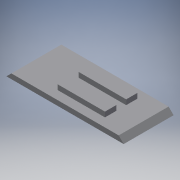
# Autodesk Inventor part: deksel token Nieuw bevestiging uitwendig
Saved by Autodesk Inventor 2018.3 (Build 223284000, 284)
## iProperties
Created: 2020-11-30
Part Number: deksel token Nieuw bevestiging uitwendig
Material: Generic
Document SubType Name: Modeling
Designer: Olivi
Density: 1 g/cm^3
Appearance: Default
Author: Olivi
Autodesk Inventor part; units mm, degrees
ref_plane "YZ Plane" through (0, 0, 0) normal (1, 0, 0) x (0, 1, 0)
ref_plane "XZ Plane" through (0, 0, 0) normal (0, 1, 0) x (-1, 0, 0)
ref_plane "XY Plane" through (0, 0, 0) normal (0, 0, 1) x (1, 0, 0)
sketch "Sketch1" plane through (0, 0, 0) normal (0, 0, 1) x (1, 0, 0)
  line L0 (0, 0) -> (43, 0)
  line L1 (43, 0) -> (43, 20)
  line L2 (43, 20) -> (0, 20)
  line L3 (0, 20) -> (0, 0)
  dimension "d0" = 43
  dimension "d1" = 20
  constraints: 8 end point, 2 parallel, 1 horizontal, 1 perpendicular
  measures "d0" distance of L2.end L1.end
  measures "d1" distance of L1.end L0.end
extrude "Extrusion1" add sketch "Sketch1" along normal blind 2
sketch "Sketch2" plane through (0, 0, 0) normal (0, -1, 0) x (1, 0, 0)
  line L0 (43, 0) -> (43, 2) projected
  line L1 (0, 0) -> (0, 2) projected
  line L2 (0, 0) -> (-2, 0)
  line L3 (-2, 0) -> (0, 2)
  line L4 (43, 0) -> (45, 0)
  line L5 (45, 0) -> (43, 2)
  dimension "d4" = 2
  dimension "d5" = 2
  constraints: 8 end point, 2 horizontal
  measures "d4" distance of L1.start L2.end
  measures "d5" distance of L0.start L4.end
extrude "Extrusion2" add sketch "Sketch2" against normal blind 20
sketch "Sketch5" plane through (0, 0, 2) normal (0, 0, 1) x (1, 0, 0)
  line L0 (15, 3.5) -> (15, 8) projected
  line L1 (34, 16.5) -> (15, 16.5) projected
  line L2 (15, 3.5) -> (34, 3.5)
  line L3 (34, 3.5) -> (34, 16.5)
  line L4 (34, 16.5) -> (15, 16.5)
  line L5 (15, 16.5) -> (15, 3.5)
  line L6 (15, 8) -> (34, 8)
  line L7 (34, 8) -> (34, 12)
  line L8 (34, 12) -> (15, 12)
  line L9 (15, 12) -> (15, 8)
  constraints: 16 end point, 4 parallel, 2 horizontal, 2 perpendicular
extrude "Extrusion5" add sketch "Sketch5" along normal blind 2 contours L0 L6 L3 L2 | L5 L1 L3 L8
body "Solid1"
